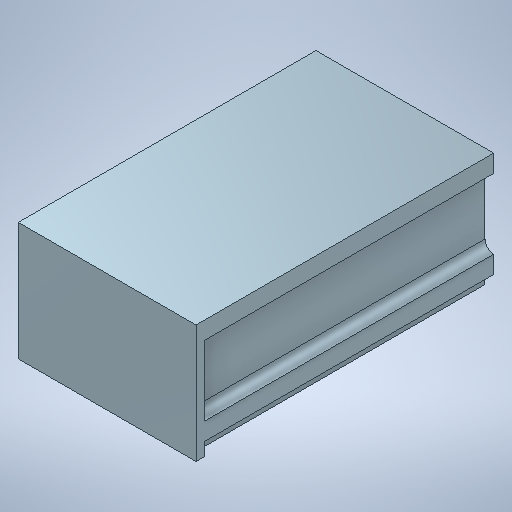
# Autodesk Inventor part: CarcasaSuperiorV2
Saved by Autodesk Inventor 2025.1 (Build 291241020, 241B)
## iProperties
Created: 2024-09-02
Part Number: CarcasaSuperiorV2
Material: Generic
Document SubType Name: Modeling
Designer: andre
Density: 1 g/cm^3
Appearance: Anodized - Blue-Gray
Author: andre
Autodesk Inventor part; units mm, degrees
ref_plane "YZ Plane" through (0, 0, 0) normal (1, 0, 0) x (0, 1, 0)
ref_plane "XZ Plane" through (0, 0, 0) normal (0, 1, 0) x (-1, 0, 0)
ref_plane "XY Plane" through (0, 0, 0) normal (0, 0, 1) x (1, 0, 0)
sketch "Sketch1" plane through (0, 0, 0) normal (0, 0, 1) x (1, 0, 0)
  line L0 (0, 0) -> (-3, 0)
  line L1 (-3, 0) -> (-3, 27)
  line L2 (-3, 27) -> (0, 27)
  line L3 (0, 21.8) -> (-2.2, 25)
  line L4 (-2.2, 25) -> (-0.6263, 25)
  line L5 (0, 1.8) -> (-2.2, 5)
  line L6 (-2.2, 5) -> (0, 5)
  line L7 (0, 27) -> (15.3, 27)
  line L8 (15.3, 27) -> (15.3, 25)
  line L9 (15.3, 25) -> (-0.6263, 25)
  line L10 (0, 21.8) -> (0, 0)
  point P0 (-1.4131, 25)
  point P1 (-1.1, 5)
  dimension "d1" = 27
  dimension "d4" = 2
  dimension "d9" = 17.5
  dimension "d10" = 2.2
  dimension "d11" = 3
  dimension "d12" = 3.2
  dimension "d23" = 20
  constraints: 22 end point, 4 parallel, 3 perpendicular, 2 horizontal, 2 horizontal alignment, 2 midpoint, 2 point on line, 1 vertical alignment
  measures "d1" distance of L0.end L1.end
  measures "d4" distance between parallel lines of L2 L4
  measures "d9" distance from line of L8 L3.end
  measures "d10" horizontal distance of L3.end L3.start
  measures "d11" distance between parallel lines of L1 L10
  measures "d12" vertical distance of L3.end L3.start
  measures "d23" distance of L5.end L3.end
extrude "Extrusion1" add sketch "Sketch1" along normal blind 66 contours L0 L1 L2 L7 L8 L9 L4 L3 L10 L6 L5
mirror "Mirror1" about plane through (15.3, 25, 0) normal (1, 0, 0) of "Extrusion1"
sketch "Sketch2" plane through (0, 0, 66) normal (0, 0, 1) x (1, 0, 0)
  line L0 (-3, 27) -> (-3, 0) projected
  line L1 (-3, 27) -> (-5, 27)
  line L2 (-5, 27) -> (-5, 23)
  line L3 (-5, 23) -> (-3, 23)
  line L4 (-3, 23) -> (-3, 27)
  line L5 (-3, 7) -> (-5, 7)
  line L6 (-5, 7) -> (-5, 3)
  line L7 (-5, 3) -> (-3, 3)
  line L8 (-3, 3) -> (-3, 7)
  line L9 (-2.2, 25) -> (32.8, 25) projected
  line L10 (-2.2, 5) -> (0, 5) projected
  point P0 (0, 0)
  point P1 (-4, 27)
  point P2 (-1.1, 5)
  dimension "d15" = 4
  dimension "d16" = 2
  dimension "d17" = 2
  dimension "d18" = 4
  dimension "d19" = 2
  constraints: 16 end point, 4 parallel, 3 point on line, 2 horizontal, 2 midpoint, 2 perpendicular
  measures "d15" distance of L1.end L2.end
  measures "d16" distance from line of point (-4, 27) L9
  measures "d17" distance from line of L5 point (-1.1, 5)
  measures "d18" distance of L5.end L6.end
  measures "d19" distance of L2.end L3.end
extrude "Extrusion2" add sketch "Sketch2" against normal up to surface (66 mm away)
fillet "Fillet1" radius 2 3 edges at (-3, 23, 33) (-3, 3, 33) (-3, 7, 33)
ref_plane "Work Plane1" through (15.3, 9, 0) normal (-1, 0, 0) x (0, 0, 1)
mirror "Mirror2" about plane through (15.3, 9, 0) normal (-1, 0, 0) of "Extrusion2", "Fillet1"
sketch "Sketch3" plane through (-2.2, 25, 0) normal (0, -1, 0) x (1, 0, 0)
  line L0 (0, 0) -> (35, 0) projected
  line L1 (35, 0) -> (35, 66) projected
  line L2 (0, 66) -> (35, 66) projected
  line L3 (0, 0) -> (0, 66) projected
  circle A0 centre (17.5, 61) radius 2.5
  circle A1 centre (17.5, 51) radius 2.5
  point P0 (2.2, 0)
  point P1 (17.5, 66)
  dimension "d24" = 5
  dimension "d26" = 15
  dimension "d27" = 5
  constraints: 2 centre point, 2 vertical alignment, 1 equal radius, 1 midpoint
  measures "d24" diameter of A0
  measures "d26" distance from line of L2 A1.centre
  measures "d27" distance from line of L2 A0.centre
extrude "Extrusion3" add sketch "Sketch3" along normal blind 15 contours A0 | A1
sketch "Sketch4" plane through (-5, 27, 66) normal (0, 1, 0) x (1, 0, 0)
  line L0 (0, 0) -> (40.6, 0)
  line L1 (40.6, 0) -> (40.6, -2)
  line L2 (40.6, -2) -> (0, -2)
  line L3 (0, -2) -> (0, 0)
  point P0 (5, 66)
  dimension "d30" = 2
  constraints: 8 end point, 2 coincident, 2 parallel, 1 horizontal, 1 perpendicular
  measures "d30" distance of L0.end L1.end
extrude "Extrusion4" add sketch "Sketch4" against normal up to surface (27 mm away)
body "Solid1"
